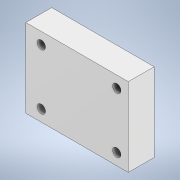
# Autodesk Inventor part: PiezaNivel
Saved by Autodesk Inventor 2021 (Build 250183000, 183)
## iProperties
Created: 2022-05-23
Part Number: PiezaNivel
Material: Plástico ABS
Document SubType Name: Modeling
Designer: 79449
Density: 1.06 g/cm^3
Appearance: Suave - Blanco
Author: 79449
Autodesk Inventor part; units mm, degrees
ref_plane "YZ Plane" through (0, 0, 0) normal (1, 0, 0) x (0, 1, 0)
ref_plane "XZ Plane" through (0, 0, 0) normal (0, 1, 0) x (-1, 0, 0)
ref_plane "XY Plane" through (0, 0, 0) normal (0, 0, 1) x (1, 0, 0)
sketch "Boceto1" plane through (0, 0, 0) normal (0, 0, 1) x (1, 0, 0)
  line L0 (-25.8, 19.8) -> (25.8, 19.8)
  line L1 (25.8, 19.8) -> (25.8, -19.8)
  line L2 (25.8, -19.8) -> (-25.8, -19.8)
  line L3 (-25.8, -19.8) -> (-25.8, 19.8)
  line L4 (-25.8, 19.8) -> (25.8, -19.8) construction
  line L5 (25.8, 19.8) -> (-25.8, -19.8) construction
  point P0 (0, 0)
  dimension "d0" = 39.6
  dimension "d1" = 51.6
  constraints: 12 end point, 2 midpoint, 2 parallel, 1 horizontal, 1 perpendicular
  measures "d0" distance of L0.end L1.end
  measures "d1" distance of L0.start L0.end
extrude "Extrusión1" add sketch "Boceto1" along normal blind 13
sketch "Boceto2" plane through (0, 0, 13) normal (0, 0, 1) x (1, 0, 0)
  circle A0 centre (-17.9984, 14) radius 2.1
  circle A1 centre (20, 14) radius 2.1
  line L0 (25.8, -19.8) -> (25.8, 19.8) projected
  line L1 (25.8, 19.8) -> (-25.8, 19.8) projected
  line L2 (-25.8, 19.8) -> (-25.8, -19.8) projected
  line L3 (20, 14) -> (-25.8, 14) construction
  line L4 (-25.8, 0) -> (25.8, 0) construction
  circle A2 centre (-17.9984, -14) radius 2.1
  circle A3 centre (20, -14) radius 2.1
  point P0 (0, 0)
  dimension "d4" = 4.2
  dimension "d5" = 4.2
  dimension "d7" = 5.8
  dimension "d8" = 5.8
  dimension "d10" = 5.8
  dimension "d11" = 7.8016
  constraints: 4 centre point, 4 end point, 2 midpoint, 2 point on line, 2 symmetric about line, 1 perpendicular, 2 other
  measures "d4" diameter of A0
  measures "d5" diameter of A1
  measures "d7" distance from line of L0 L3.start
  measures "d8" distance from line of L1 L3.start
  measures "d10" distance from line of L1 A0.centre
  measures "d11" distance from line of L2 A0.centre
extrude "Extrusión2" cut sketch "Boceto2" against normal through all
